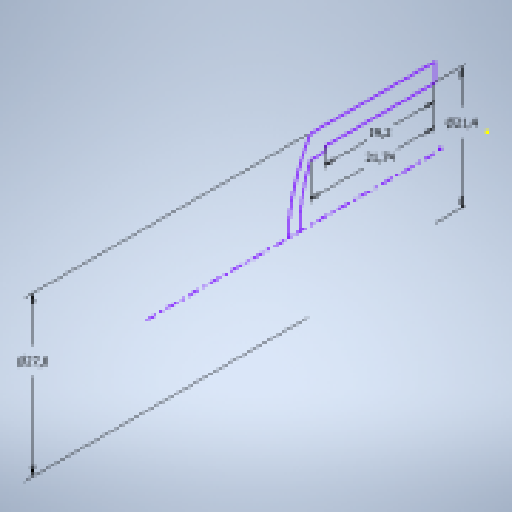
# Autodesk Inventor part: TapaPVC
Saved by Autodesk Inventor 2023.1 (Build 271208000, 208)
## iProperties
Created: 2022-08-28
Part Number: TapaPVC
Material: Generic
Document SubType Name: Modeling
Designer: Daniel Peña
Density: 1 g/cm^3
Appearance: Default
Author: Daniel Peña
Autodesk Inventor part; units mm, degrees
ref_plane "YZ Plane" through (0, 0, 0) normal (1, 0, 0) x (0, 1, 0)
ref_plane "XZ Plane" through (0, 0, 0) normal (0, 1, 0) x (-1, 0, 0)
ref_plane "XY Plane" through (0, 0, 0) normal (0, 0, 1) x (1, 0, 0)
sketch "Sketch1" plane through (0, 0, 0) normal (1, 0, 0) x (0, 1, 0)
  line L0 (1.4408, 9.2852) -> (1.4408, 59.8704)
  line L1 (15.3408, 9.2852) -> (15.3408, 31.0252)
  line L2 (12.1408, 9.2852) -> (12.1408, 28.4852)
  line L3 (12.1408, 28.4852) -> (11.3041, 28.4852)
  line L4 (11.3041, 28.4852) -> (11.3041, 31.0252)
  arc A0 (15.3408, 31.0252) -> (1.4408, 34.8852) centre (1.538, 8.2778) ccw
  arc A1 (11.3041, 31.0252) -> (1.4408, 33.0328) centre (1.538, 8.2778) ccw
  line L5 (12.1408, 9.2852) -> (15.3408, 9.2852)
  line L6 (1.4408, 34.8852) -> (1.4408, 33.0328)
  point P0 (0, 0)
  point P1 (1.4408, 33.0328)
  dimension "d1" = 27.8
  dimension "d3" = 19.2
  dimension "d4" = 21.74
  dimension "d5" = 21.4
  dimension "d6" = 25.6
  constraints: 14 end point, 4 point on circle, 3 vertical, 2 centre point, 2 horizontal, 1 collinear, 1 perpendicular, 1 point on line
  measures "d1" diameter of L1 L0
  measures "d3" distance of L2.start L2.end
  measures "d4" vertical distance of L4.end L2.start
  measures "d5" diameter of L2 L0
  measures "d6" distance from line of L5 L6.start
revolve "Revolution1" add sketch "Sketch1" angle 360 about axis through (0, 1.4408, 9.2852) along (0, 0, 1)
sketch "Sketch2" plane through (0, 1.4408, 9.2852) normal (0, 0, -1) x (-1, 0, 0)
  circle A0 centre (0, 0) radius 15.65 construction
  line L0 (0, 15.65) -> (11.0662, 11.0662)
  line L1 (11.0662, 11.0662) -> (15.65, 0)
  line L2 (15.65, 0) -> (11.0662, -11.0662)
  line L3 (11.0662, -11.0662) -> (0, -15.65)
  line L4 (0, -15.65) -> (-11.0662, -11.0662)
  line L5 (-11.0662, -11.0662) -> (-15.65, 0)
  line L6 (-15.65, 0) -> (-11.0662, 11.0662)
  line L7 (-11.0662, 11.0662) -> (0, 15.65)
  circle A1 centre (0, 0) radius 13.9
  point P0 (0, -1.4408)
  dimension "d8" = 31.3
  constraints: 16 end point, 2 coincident, 1 centre point, 1 vertical alignment, 19 other
extrude "Extrusion1" add sketch "Sketch2" against normal blind 5
body "Solid1"
